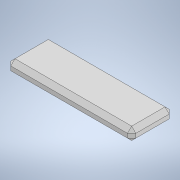
# Autodesk Inventor part: Battery
Saved by Autodesk Inventor 2020 (Build 240168000, 168)
## iProperties
Created: 2022-02-24
Part Number: Battery
Material: Типовые
Document SubType Name: Modeling
Designer: NoName
Density: 1 g/cm^3
Appearance: По умолчанию
Author: NoName
Autodesk Inventor part; units mm, degrees
ref_plane "YZ Plane" through (0, 0, 0) normal (1, 0, 0) x (0, 1, 0)
ref_plane "XZ Plane" through (0, 0, 0) normal (0, 1, 0) x (-1, 0, 0)
ref_plane "XY Plane" through (0, 0, 0) normal (0, 0, 1) x (1, 0, 0)
sketch "Эскиз1" plane through (0, 0, 0) normal (0, 1, 0) x (-1, 0, 0)
  line L0 (-15, -5) -> (15, -5)
  line L1 (15, -5) -> (15, 5)
  line L2 (15, 5) -> (-15, 5)
  line L3 (-15, 5) -> (-15, -5)
  point P0 (0, 0)
  point P1 (-15, 0)
  point P2 (0, -5)
  dimension "d0" = 10
  dimension "d1" = 30
  constraints: 8 end point, 2 midpoint, 2 parallel, 1 horizontal, 1 horizontal alignment, 1 perpendicular, 1 vertical alignment
  measures "d0" distance between parallel lines of L2 L0
  measures "d1" distance between parallel lines of L1 L3
extrude "Выдавливание1" add sketch "Эскиз1" along normal blind 3
chamfer "Фаска1" distance 1 angle 45 12 edges at (-15, 3, 0) (-15, 0, 0) (0, 3, 5) (0, 0, 5) (15, 1.5, 5) (15, 3, 0) (15, 0, 0) (15, 1.5, -5) (0, 3, -5) (0, 0, -5) (-15, 1.5, -5) (-15, 1.5, 5)
